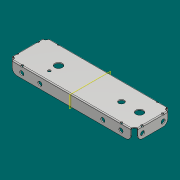
# Autodesk Inventor part: back
Saved by Autodesk Inventor 2018.2 (Build 222227000, 227)
## iProperties
Created: 2019-11-16
Part Number: back
Material: アルミニウム 6061
Document SubType Name: Sheet Metal
Designer: gisen
Density: 2.7 g/cm^3
Sheet Metal Rule: Default_mm
Appearance: アルミニウム - フラット
Author: gisen
Autodesk Inventor part; units mm, degrees
ref_plane "XZ Plane" through (0, 0, 0) normal (0, 1, 0) x (-1, 0, 0)
ref_plane "XY Plane" through (0, 0, 0) normal (0, 0, 1) x (1, 0, 0)
sketch "スケッチ1" plane through (0, 0, 0) normal (0, 0, 1) x (1, 0, 0)
  line L0 (-67.5, -20) -> (67.5, -20)
  line L1 (67.5, -20) -> (67.5, 20)
  line L2 (67.5, 20) -> (-67.5, 20)
  line L3 (-67.5, 20) -> (-67.5, -20)
  line L4 (-67.5, -20) -> (67.5, 20) construction
  line L5 (67.5, -20) -> (-67.5, 20) construction
  line L6 (-67.5, 16) -> (-63.5, 16)
  line L7 (-63.5, 16) -> (-63.5, 20)
  line L8 (-67.5, -16) -> (-63.5, -16)
  line L9 (-63.5, -16) -> (-63.5, -20)
  line L10 (63.5, 20) -> (63.5, 16)
  line L11 (63.5, 16) -> (67.5, 16)
  line L12 (67.5, -16) -> (63.5, -16)
  line L13 (63.5, -16) -> (63.5, -20)
  point P0 (0, 0)
  dimension "d0" = 135
  dimension "d1" = 40
  dimension "d2" = 4
  measures "d0" distance of L1.end L2.end
  measures "d1" distance of L0.end L1.end
  measures "d2" distance of L6.end L7.end
extrude "プレート1" add sketch "スケッチ1" along normal blind 1 contours L9 L8 L3 L6 L7 L2 L10 L11 L1 L12 L13 L0
sketch "スケッチ2" plane through (63.5, 19, 1) normal (0, 1, 0) x (-1, 0, 0)
  line L0 (127, 0) -> (0, 0)
  line L1 (0, 0) -> (0, -12)
  line L2 (0, -12) -> (127, -12)
  line L3 (127, -12) -> (127, 0)
  constraints: 6 end point, 1 horizontal, 1 perpendicular, 1 vertical
edge flange "フランジ1" height 12 angle 90 thickness 1 bend radius 0 thickness toward (0, 1, 0) relief straight relief width 1 relief depth 0.5 corner gap 0 corner form 0 edges at (0, 20, 0) (0, -20, 0) (67.5, 0, 0) (-67.5, 0, 0) wall of the first edge with corners at (-63.5, 19, 1) (63.5, 19, 1) (63.5, 19, -11) (-63.5, 19, -11)
bend "曲げ1"
corner "コーナー1"
sketch "スケッチ3" plane through (-63.5, 20, -11) normal (0, 1, 0) x (1, 0, 0)
  line L0 (0, 0) -> (127, 0) construction
  line L1 (127, -12) -> (0, -12) construction
  line L2 (127, 0) -> (0, 0) construction
  line L3 (63.5, 0) -> (63.5, -12) construction
  line L4 (0, -12) -> (127, -12) construction
  line L5 (63.5, -5) -> (29.75, -5) construction
  line L6 (29.75, -5) -> (10.25, -5) construction
  circle A0 centre (10.25, -5) radius 2.25
  circle A1 centre (29.75, -5) radius 2.25
  circle A2 centre (116.75, -5) radius 2.25
  circle A3 centre (97.25, -5) radius 2.25
  point P0 (63.5, -11)
  dimension "d14" = 33.75
  dimension "d15" = 7
  dimension "d16" = 19.5
  dimension "d17" = 4.5
  constraints: 6 end point, 4 centre point, 2 coincident, 2 horizontal, 2 midpoint, 2 symmetric about line, 1 equal radius, 1 point on line, 2 other
  measures "d14" distance of L5.start L5.end
  measures "d15" distance between parallel lines of L1 L5
  measures "d16" distance of L5.end L6.end
  measures "d17" diameter of A0
extrude "押し出し1" cut sketch "スケッチ3" against normal through all
fillet "フィレット1" radius 5 4 edges at (-63.5, 19.5, -11) (63.5, 19.5, -11) (63.5, -19.5, -11) (-63.5, -19.5, -11)
sketch "スケッチ4" plane through (67.5, -16, -11) normal (1, 0, 0) x (0, 0, -1)
  line L0 (0, 32) -> (0, 0) construction
  line L1 (-12, 0) -> (-12, 32) construction
  line L2 (-12, 16) -> (0, 16) construction
  line L3 (-5, 22) -> (-5, 0) construction
  circle A0 centre (-5, 27) radius 2.25
  line L4 (-10.999, 32) -> (0, 32) projected
  circle A1 centre (-5, 5) radius 2.25
  point P0 (-11, 16)
  dimension "d21" = 7
  dimension "d22" = 16
  dimension "d23" = 5
  dimension "d24" = 4.5
  constraints: 4 end point, 2 centre point, 2 midpoint, 1 point on line, 1 symmetric about line, 1 vertical, 2 other
  measures "d21" distance between parallel lines of L1 L3
  measures "d22" distance of the line from the sketch origin of L2
  measures "d24" diameter of A0
extrude "押し出し2" cut sketch "スケッチ4" against normal through all
fillet "フィレット2" radius 5 4 edges at (67, 16, -11) (67, -16, -11) (-67, 16, -11) (-67, -16, -11)
sketch "スケッチ5" plane through (0, 0, 1) normal (0, 0, 1) x (1, 0, 0)
  line L0 (-66.499, 16) -> (-66.499, -16) construction
  line L1 (-63.5, -16) -> (-66.499, -16) construction
  line L2 (-63.5, -18.999) -> (-63.5, -16) construction
  line L3 (-63.5, -18.999) -> (63.5, -18.999) construction
  line L4 (63.5, -16) -> (63.5, -18.999) construction
  line L5 (66.499, -16) -> (63.5, -16) construction
  line L6 (66.499, -16) -> (66.499, 16) construction
  line L7 (63.5, 16) -> (66.499, 16) construction
  line L8 (63.5, 18.999) -> (63.5, 16) construction
  line L9 (63.5, 18.999) -> (-63.5, 18.999) construction
  line L10 (-63.5, 16) -> (-63.5, 18.999) construction
  line L11 (-66.499, 16) -> (-63.5, 16) construction
  circle A0 centre (33.75, 0) radius 3.05
  line L12 (-66.499, 0) -> (66.499, 0) construction
  circle A1 centre (53.25, 0) radius 4.05
  point P0 (0, 0)
  dimension "d28" = 6.1
  dimension "d29" = 33.75
  dimension "d30" = 8.1
  dimension "d31" = 53.25
  constraints: 2 centre point, 2 end point, 2 midpoint, 2 point on line
  measures "d28" diameter of A0
  measures "d29" distance of point (0, 0) A0.centre
  measures "d30" diameter of A1
  measures "d31" distance of A1.centre point (0, 0)
extrude "押し出し3" cut sketch "スケッチ5" against normal through all
fillet "フィレット3" radius 2.5 4 edges at (63.5, -16, 0.5) (63.5, 16, 0.5) (-63.5, 16, 0.5) (-63.5, -16, 0.5)
unfold all bends "展開1" k factor 0.44 fixed face at (-32.2651, 0, 1)
sketch "スケッチ6" plane through (0, 0, 1) normal (0, 0, 1) x (1, 0, 0)
  line L0 (-63.5, 19.6917) -> (63.5, 19.6917) construction
  line L1 (-63.5, 18.999) -> (-63.5, 19.6917) construction
  line L2 (63.5, 18.999) -> (-63.5, 18.999) construction
  line L3 (63.5, 19.6917) -> (63.5, 18.999) construction
  line L4 (-67.1917, -16) -> (-67.1917, 16) construction
  line L5 (-66.499, -16) -> (-67.1917, -16) construction
  line L6 (-66.499, 16) -> (-66.499, -16) construction
  line L7 (-67.1917, 16) -> (-66.499, 16) construction
  line L8 (-66.499, 0) -> (66.499, 0) construction
  line L9 (66.499, -16) -> (66.499, 16) construction
  line L10 (-63.5, 18.999) -> (63.5, 18.999) construction
  line L11 (0, 18.999) -> (0, -18.999) construction
  line L12 (-63.5, -18.999) -> (63.5, -18.999) construction
  line L13 (-67.1917, 16) -> (-66.499, 16) construction
  line L14 (-66.8454, 16) -> (-66.8454, -16) construction
  line L15 (-63.5, 19.6917) -> (-63.5, 18.999) construction
  line L16 (-63.5, 19.3454) -> (63.5, 19.3454) construction
  line L17 (63.5, 19.6917) -> (63.5, 18.999) construction
  circle A0 centre (-73.1907, 11) radius 2.25 construction
  line L18 (-73.1907, 11) -> (-66.8454, 11) construction
  circle A1 centre (-53.25, 25.6907) radius 2.25 construction
  line L19 (-53.25, 25.6907) -> (-53.25, 19.3454) construction
  circle A2 centre (-53.25, 19.3454) radius 1.1
  circle A3 centre (-66.8454, 11) radius 1.1
  circle A4 centre (-53.25, -19.3454) radius 1.1
  circle A5 centre (-66.8454, -11) radius 1.1
  circle A6 centre (53.25, 19.3454) radius 1.1
  circle A7 centre (66.8454, 11) radius 1.1
  circle A8 centre (66.8454, -11) radius 1.1
  circle A9 centre (53.25, -19.3454) radius 1.1
  point P0 (0, 0)
  dimension "d35" = 2.2
  constraints: 12 end point, 8 centre point, 8 midpoint, 6 symmetric about line, 2 coincident, 2 point on line, 1 equal radius, 1 parallel, 1 perpendicular, 6 other
  measures "d35" diameter of A2
extrude "押し出し4" cut sketch "スケッチ6" against normal up to surface (1 mm away)
refold all bends "再折り曲げ1"
sketch "スケッチ7" plane through (0, 0, 1) normal (0, 0, 1) x (1, 0, 0)
  circle A0 centre (-33.75, 0) radius 4.1
  circle A1 centre (-33.75, -10) radius 1.55
  line L0 (-67.5, -9.956) -> (-67.5, 9.956) projected
  line L1 (0, 0) -> (-42.5, 0) construction
  line L2 (-33.75, -10) -> (-33.75, 0) construction
  dimension "d38" = 8.2
  dimension "d39" = 3.1
  dimension "d41" = 33.75
  dimension "d42" = 67.5
  dimension "d45" = 10
  dimension "d47" = 90
  constraints: 4 end point, 2 centre point, 1 horizontal, 1 point on line
  measures "d38" diameter of A0
  measures "d39" diameter of A1
  measures "d41" distance of L1.start L2.end
  measures "d42" distance from line of L0 L1.start
  measures "d45" distance of L2.start L2.end
  measures "d47" angle of L2 L1
extrude "押し出し5" cut sketch "スケッチ7" against normal through all
equation "\"d3\" = Thickness"
equation "\"d4\" = BendReliefWidth"
equation "\"d5\" = BendReliefDepth"
equation "\"d6\" = MinimumRemnant"
equation "\"d11\" = CornerReliefSize"
equation "\"d12\" = GapSize"
equation "\"BendReliefWidth\" = Thickness"
equation "\"BendReliefDepth\" = 0.5 * Thickness"
equation "\"CornerReliefSize\" = 4 * Thickness"
equation "\"MinimumRemnant\" = 2 * Thickness"
equation "\"GapSize\" = Thickness"
equation "\"Thickness\" = 1"
